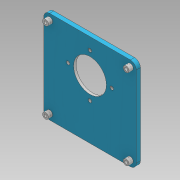
# Autodesk Inventor part: 연결부
Saved by Autodesk Inventor 2018 (Build 220112000, 112)
## iProperties
Created: 2018-04-05
Part Number: 연결부
Material: 일반
Document SubType Name: Modeling
Designer: CK
Density: 1 g/cm^3
Appearance: 기본값
Mass: 51.2428 g
Surface Area: 256.646 cm^2
Volume: 51.2428 cm^3
Author: CK
Autodesk Inventor part; units mm, degrees
ref_plane "YZ Plane" through (0, 0, 0) normal (1, 0, 0) x (0, 1, 0)
ref_plane "XZ Plane" through (0, 0, 0) normal (0, 1, 0) x (-1, 0, 0)
ref_plane "XY Plane" through (0, 0, 0) normal (0, 0, 1) x (1, 0, 0)
sketch "스케치1" plane through (0, 0, 0) normal (0, 1, 0) x (-1, 0, 0)
  line L0 (-55, 55) -> (55, 55)
  line L1 (55, 55) -> (55, -55)
  line L2 (55, -55) -> (-55, -55)
  line L3 (-55, -55) -> (-55, 55)
  line L4 (-55, 55) -> (55, -55) construction
  line L5 (55, 55) -> (-55, -55) construction
  point P0 (0, 0)
  dimension "d0" = 110
  dimension "d1" = 110
  constraints: 12 end point, 2 midpoint, 2 parallel, 1 horizontal, 1 perpendicular
  measures "d0" distance of L1.end L2.end
  measures "d1" distance of L0.end L1.end
extrude "돌출1" add sketch "스케치1" along normal blind 5
fillet "모깎기1" radius 7 1 edges at (55, 2.5, 55)
fillet "모깎기2" radius 7 3 edges at (55, 2.5, -55) (-55, 2.5, -55) (-55, 2.5, 55)
sketch "스케치5" plane through (0, 0, 0) normal (0, -1, 0) x (1, 0, 0)
  arc A0 (55, 48) -> (48, 55) centre (48, 48) ccw projected
  circle A1 centre (48, 48) radius 3.5
  point P0 (0, 0)
  dimension "d15" = 7
  constraints: 1 centre point, 1 coincident
  measures "d15" diameter of A1
extrude "돌출5" add sketch "스케치5" along normal blind 5
mirror "미러1" about plane through (0, 0, 0) normal (1, 0, 0) of "돌출5"
mirror "미러2" about plane through (0, 0, 0) normal (0, 0, 1) of "돌출5", "미러1"
sketch "스케치6" plane through (0, 5, 0) normal (0, 1, 0) x (1, 0, 0)
  arc A0 (-55, -48) -> (-48, -55) centre (-48, -48) ccw projected
  arc A1 (-48, 55) -> (-55, 48) centre (-48, 48) ccw projected
  arc A2 (55, 48) -> (48, 55) centre (48, 48) ccw projected
  arc A3 (48, -55) -> (55, -48) centre (48, -48) ccw projected
  circle A4 centre (-48, -48) radius 3.25
  point P0 (0, 0)
  dimension "d18" = 6.5
  constraints: 1 centre point, 1 coincident
  measures "d18" diameter of A4
extrude "돌출6" cut sketch "스케치6" against normal blind 7
mirror "미러3" about plane through (0, 0, 0) normal (1, 0, 0) of "돌출6"
mirror "미러4" about plane through (0, 0, 0) normal (0, 0, 1) of "돌출6", "미러3"
sketch "스케치7" plane through (-48, -2, 48) normal (0, 1, 0) x (1, 0, 0)
  arc A0 (-7, 0) -> (0, -7) centre (0, 0) ccw projected
  circle A1 centre (0, 0) radius 1.8
  point P0 (48, 48)
  dimension "d21" = 3.6
  constraints: 1 centre point, 1 coincident
  measures "d21" diameter of A1
extrude "돌출7" cut sketch "스케치7" against normal through all
mirror "미러5" about plane through (0, 0, 0) normal (0, 0, 1) of "돌출7"
mirror "미러6" about plane through (0, 0, 0) normal (1, 0, 0) of "돌출7", "미러5"
sketch "스케치9" plane through (0, 5, 0) normal (0, 1, 0) x (1, 0, 0)
  circle A0 centre (0, -15) radius 32.5
  line L0 (42.9638, 0) -> (-42.9638, 0) construction
  point P0 (0, 0)
  dimension "d32" = 65
  dimension "d33" = 15
  constraints: 2 end point, 1 centre point, 1 horizontal
  measures "d32" diameter of A0
  measures "d33" distance from line of L0 A0.centre
extrude "돌출9" cut sketch "스케치9" against normal blind 1
sketch "스케치10" plane through (0, 4, 15) normal (0, 1, 0) x (1, 0, 0)
  circle A0 centre (0, 0) radius 22.5
  point P0 (0, 15)
  dimension "d36" = 45
  constraints: 1 centre point
  measures "d36" diameter of A0
extrude "돌출10" cut sketch "스케치10" against normal blind 1
sketch "스케치11" plane through (0, 3, 15) normal (0, 1, 0) x (1, 0, 0)
  circle A0 centre (0, 0) radius 19.5
  point P0 (0, 15)
  dimension "d39" = 39
  constraints: 1 centre point
  measures "d39" diameter of A0
extrude "돌출11" cut sketch "스케치11" against normal through all
chamfer "모따기2" distance 1 angle 45 1 edges at (-22.5, 4, 15)
sketch "스케치12" plane through (0, 4, 15) normal (0, 1, 0) x (1, 0, 0)
  circle A0 centre (0, 0) radius 26 construction
  circle A1 centre (0, -26) radius 2
  point P0 (0, 15)
  dimension "d48" = 52
  dimension "d49" = 4
  constraints: 1 centre point, 1 vertical alignment, 2 other
  measures "d49" diameter of A1
extrude "돌출12" cut sketch "스케치12" against normal blind 10
pattern_circular "원형 패턴1" count 4 over 360 about axis through (0, 3.5, 15) along (0, 1, 0) of "돌출12"
